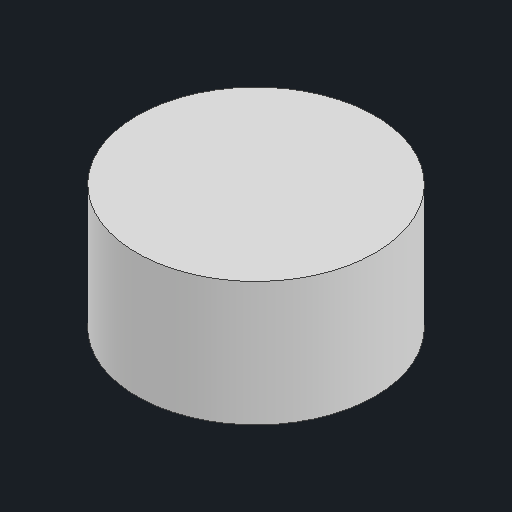
# Autodesk Inventor part: 큰베어링 정렬
Saved by Autodesk Inventor 2027.1 (Build 311270010, 270A)
## iProperties
Created: 2026-08-22
Part Number: 큰베어링 정렬
Material: 일반
Document SubType Name: Modeling
Designer: moieboy9999
Density: 1 g/cm^3
Appearance: 기본값
Mass: 0.623213 g
Surface Area: 4.24508 cm^2
Volume: 0.623213 cm^3
Author: moieboy9999
## iProperties of the stored document 큰베어링 정렬_3D 인쇄.ipt
Created: 2026-08-22
Part Number: 큰베어링 정렬_3D 인쇄
Material: 일반
Document SubType Name: Modeling
Designer: maker
Density: 1 g/cm^3
Appearance: 기본값
Author: maker
Autodesk Inventor part; units mm, degrees
ref_plane "YZ Plane" through (0, 0, 0) normal (1, 0, 0) x (0, 1, 0)
ref_plane "XZ Plane" through (0, 0, 0) normal (0, 1, 0) x (-1, 0, 0)
ref_plane "XY Plane" through (0, 0, 0) normal (0, 0, 1) x (1, 0, 0)
sketch "스케치1" plane through (0, 0, 0) normal (0, 1, 0) x (-1, 0, 0)
  circle A0 centre (0, 0) radius 5.75
  dimension "d0" = 11.5
  constraints: 1 centre point, 1 coincident
  measures "d0" diameter of A0
extrude "돌출1" add sketch "스케치1" along normal blind 1
move faces "이동1" translate (0, 5, 0) faces at (-0.1148, 1, 1.5963)
